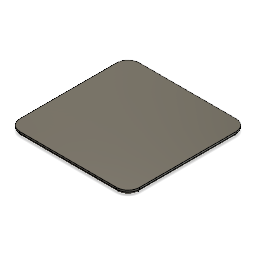
bottom (Autodesk Fusion 360 design; units mm, degrees)
Autodesk Fusion 360 part; units mm, degrees
sketch "Sketch1" plane through (0, 0, 0) normal (0, 1, 0) x (1, 0, 0)
  line L0 (35.25, -35.25) -> (-35.25, -35.25)
  line L1 (-35.25, -35.25) -> (-35.25, 35.25)
  line L2 (-35.25, 35.25) -> (35.25, 35.25)
  line L3 (35.25, 35.25) -> (35.25, -35.25)
  line L4 (35.25, -35.25) -> (-35.25, 35.25) construction
  line L5 (-35.25, -35.25) -> (35.25, 35.25) construction
  dimension "d1" = 70.5
  dimension "d2" = 70.5
  constraint perpendicular L0 L1
  constraint parallel L0 L2
  constraint parallel L1 L3
  constraint horizontal L0
  constraint coincident L4 origin
  constraint coincident L5 origin
  measures "d1" distance of L1.end L2.end
  measures "d2" distance of L0.end L1.end
extrude "Extrude1" add sketch "Sketch1" along normal blind 2
fillet "Fillet1" radius 6.75 4 edges at (-35.25, 1, 35.25) (-35.25, 1, -35.25) (35.25, 1, 35.25) (35.25, 1, -35.25)
fillet "Fillet2" radius 2 8 edges at (0, 0, -35.25) (-33.273, 0, -33.273) (-35.25, 0, 0) (-33.273, 0, 33.273) (0, 0, 35.25) (33.273, 0, 33.273) (35.25, 0, 0) (33.273, 0, -33.273)
extrude "Extrude2" add 1 faces at (9.5, 2, 11.75) along direction (0, 1, 0) blind 1
